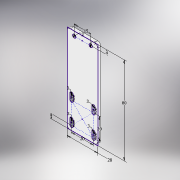
# Autodesk Inventor part: EncoderPCBMount
Saved by Autodesk Inventor 2018 (Build 220112000, 112)
## iProperties
Created: 2018-03-25
Part Number: EncoderPCBMount
Material: ABS Plastic
Document SubType Name: Modeling
Designer: mansu
Density: 1.06 g/cm^3
Appearance: Smooth - White
Author: mansu
Autodesk Inventor part; units mm, degrees
ref_plane "YZ Plane" through (0, 0, 0) normal (1, 0, 0) x (0, 1, 0)
ref_plane "XZ Plane" through (0, 0, 0) normal (0, 1, 0) x (-1, 0, 0)
ref_plane "XY Plane" through (0, 0, 0) normal (0, 0, 1) x (1, 0, 0)
sketch "Sketch1" plane through (0, 0, 0) normal (0, 1, 0) x (-1, 0, 0)
  line L0 (0, 0) -> (-28, 0)
  line L1 (-28, 0) -> (-28, -80)
  line L2 (-28, -80) -> (0, -80)
  line L3 (0, -80) -> (0, 0)
  line L4 (-4, -56) -> (-24, -56) construction
  line L5 (-24, -56) -> (-24, -76) construction
  line L6 (-24, -76) -> (-4, -76) construction
  line L7 (-4, -76) -> (-4, -56) construction
  line L8 (-4, -56) -> (-24, -76) construction
  line L9 (-24, -56) -> (-4, -76) construction
  line L10 (-4, -76) -> (-4, -71) construction
  line L11 (-2.5, -76) -> (-2.5, -71)
  line L12 (-5.5, -71) -> (-5.5, -76)
  arc A0 (-5.5, -76) -> (-2.5, -76) centre (-4, -76) ccw
  arc A1 (-2.5, -71) -> (-5.5, -71) centre (-4, -71) ccw
  line L13 (-24, -76) -> (-24, -71) construction
  line L14 (-22.5, -76) -> (-22.5, -71)
  line L15 (-25.5, -71) -> (-25.5, -76)
  arc A2 (-25.5, -76) -> (-22.5, -76) centre (-24, -76) ccw
  arc A3 (-22.5, -71) -> (-25.5, -71) centre (-24, -71) ccw
  line L16 (-4, -56) -> (-4, -51) construction
  line L17 (-2.5, -56) -> (-2.5, -51)
  line L18 (-5.5, -51) -> (-5.5, -56)
  arc A4 (-5.5, -56) -> (-2.5, -56) centre (-4, -56) ccw
  arc A5 (-2.5, -51) -> (-5.5, -51) centre (-4, -51) ccw
  line L19 (-24, -56) -> (-24, -51) construction
  line L20 (-22.5, -56) -> (-22.5, -51)
  line L21 (-25.5, -51) -> (-25.5, -56)
  arc A6 (-25.5, -56) -> (-22.5, -56) centre (-24, -56) ccw
  arc A7 (-22.5, -51) -> (-25.5, -51) centre (-24, -51) ccw
  circle A8 centre (-6.5, -4) radius 1.5
  circle A9 centre (-21.5, -4) radius 1.5
  line L22 (-6.5, -4) -> (-21.5, -4) construction
  point P0 (-14, -66)
  point P1 (-14, -66)
  point P2 (-14, -80)
  point P3 (-4, -73.5)
  point P4 (-24, -73.5)
  point P5 (-4, -53.5)
  point P6 (-24, -53.5)
  point P7 (-14, -4)
  point P8 (-14, 0)
  dimension "d0" = 80
  dimension "d1" = 28
  dimension "d2" = 20
  dimension "d3" = 20
  dimension "d4" = 4
  dimension "d5" = 5
  dimension "d6" = 3
  dimension "d7" = 5
  dimension "d8" = 3
  dimension "d9" = 5
  dimension "d10" = 3
  dimension "d11" = 5
  dimension "d12" = 3
  dimension "d16" = 3
  dimension "d17" = 3
  dimension "d18" = 15
  dimension "d19" = 4
  constraints: 54 end point, 16 point on circle, 16 tangent, 10 centre point, 10 midpoint, 9 parallel, 3 horizontal, 3 point on line, 2 perpendicular, 2 vertical alignment, 1 horizontal alignment
  measures "d0" distance of L0.end L1.end
  measures "d1" distance of L1.end L2.end
  measures "d2" distance of L6.end L5.end
  measures "d3" distance of L5.end L4.end
  measures "d4" distance between parallel lines of L2 L6
  measures "d5" distance of L6.end L10.end
  measures "d6" diameter of A1
  measures "d7" distance of L5.end L13.end
  measures "d8" diameter of A3
  measures "d9" distance of L4.start L16.end
  measures "d10" diameter of A5
  measures "d11" distance of L4.end L19.end
  measures "d12" diameter of A7
  measures "d16" diameter of A8
  measures "d17" diameter of A9
  measures "d18" distance of L22.end L22.start
  measures "d19" distance between parallel lines of L0 L22
extrude "Extrusion1" add sketch "Sketch1" along normal blind 3 contours L3 L2 L1 L0 | A8 | A9
fillet "Fillet1" radius 3 4 edges at (0, 1.5, 0) (28, 1.5, 0) (0, 1.5, -80) (28, 1.5, -80)
extrude "Extrusion2" cut sketch "Sketch1" along normal through all contours A8 | A9
body "Solid1"
